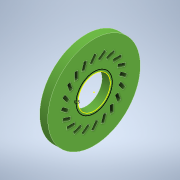
# Autodesk Inventor part: encoder
Saved by Autodesk Inventor 2021 (Build 250183000, 183)
## iProperties
Created: 2021-12-11
Part Number: encoder
Material: Generic
Document SubType Name: Modeling
Designer: Juan M. Casillas
Density: 1 g/cm^3
Appearance: Default
Author: Juan M. Casillas
Autodesk Inventor part; units mm, degrees
ref_plane "YZ Plane" through (0, 0, 0) normal (1, 0, 0) x (0, 1, 0)
ref_plane "XZ Plane" through (0, 0, 0) normal (0, 1, 0) x (-1, 0, 0)
ref_plane "XY Plane" through (0, 0, 0) normal (0, 0, 1) x (1, 0, 0)
sketch "Sketch1" plane through (0, 0, 0) normal (1, 0, 0) x (0, 1, 0)
  circle A0 centre (0, 0) radius 4
  circle A1 centre (0, 0) radius 11.5
  dimension "d0" = 8
  dimension "d1" = 23
  constraints: 2 centre point, 2 coincident
  measures "d0" diameter of A0
  measures "d1" diameter of A1
extrude "Extrusion1" add sketch "Sketch1" along normal mid plane 2
sketch "Sketch2" plane through (1, 0, 0) normal (1, 0, 0) x (0, 0, -1)
  circle A0 centre (0, 0) radius 4 projected
  circle A1 centre (0, 0) radius 4.5
  dimension "d4" = 0.5
  constraints: 1 centre point
  measures "d4" radial gap between concentric circles of A0 A1
sketch "Sketch3" plane through (1, 0, 0) normal (1, 0, 0) x (0, 0, -1)
  circle A0 centre (0, 0) radius 11.5 construction
  circle A1 centre (0, 0) radius 4.5 construction
  line L0 (-4.413, 10.6196) -> (-4.413, 0.8804) construction
  line L1 (-4.813, 6.75) -> (-4.013, 6.75)
  line L2 (-4.013, 6.75) -> (-4.013, 4.75)
  line L3 (-4.013, 4.75) -> (-4.813, 4.75)
  line L4 (-4.813, 4.75) -> (-4.813, 6.75)
  line L5 (-4.813, 6.75) -> (-4.013, 4.75) construction
  line L6 (-4.013, 6.75) -> (-4.813, 4.75) construction
  line L7 (-5.2844, 3.2774) -> (-6.0453, 3.0302)
  line L8 (-6.6633, 4.9323) -> (-5.2844, 3.2774) construction
  line L9 (-5.9025, 5.1795) -> (-6.0453, 3.0302) construction
  line L10 (-6.0453, 3.0302) -> (-6.6633, 4.9323)
  line L11 (-6.6633, 4.9323) -> (-5.9025, 5.1795)
  line L12 (-5.9025, 5.1795) -> (-5.2844, 3.2774)
  line L13 (-6.0386, 1.484) -> (-6.6858, 1.0138)
  line L14 (-7.8614, 2.6318) -> (-6.0386, 1.484) construction
  line L15 (-7.2142, 3.1021) -> (-6.6858, 1.0138) construction
  line L16 (-6.6858, 1.0138) -> (-7.8614, 2.6318)
  line L17 (-7.8614, 2.6318) -> (-7.2142, 3.1021)
  line L18 (-7.2142, 3.1021) -> (-6.0386, 1.484)
  line L19 (-6.2016, -0.4546) -> (-6.6719, -1.1018)
  line L20 (-8.2899, 0.0737) -> (-6.2016, -0.4546) construction
  line L21 (-7.8197, 0.7209) -> (-6.6719, -1.1018) construction
  line L22 (-6.6719, -1.1018) -> (-8.2899, 0.0737)
  line L23 (-8.2899, 0.0737) -> (-7.8197, 0.7209)
  line L24 (-7.8197, 0.7209) -> (-6.2016, -0.4546)
  line L25 (-5.7576, -2.3488) -> (-6.0048, -3.1096)
  line L26 (-7.9069, -2.4916) -> (-5.7576, -2.3488) construction
  line L27 (-7.6597, -1.7308) -> (-6.0048, -3.1096) construction
  line L28 (-6.0048, -3.1096) -> (-7.9069, -2.4916)
  line L29 (-7.9069, -2.4916) -> (-7.6597, -1.7308)
  line L30 (-7.6597, -1.7308) -> (-5.7576, -2.3488)
  line L31 (-4.75, -4.013) -> (-4.75, -4.813)
  line L32 (-6.75, -4.813) -> (-4.75, -4.013) construction
  line L33 (-6.75, -4.013) -> (-4.75, -4.813) construction
  line L34 (-4.75, -4.813) -> (-6.75, -4.813)
  line L35 (-6.75, -4.813) -> (-6.75, -4.013)
  line L36 (-6.75, -4.013) -> (-4.75, -4.013)
  line L37 (-3.2774, -5.2844) -> (-3.0302, -6.0453)
  line L38 (-4.9323, -6.6633) -> (-3.2774, -5.2844) construction
  line L39 (-5.1795, -5.9025) -> (-3.0302, -6.0453) construction
  line L40 (-3.0302, -6.0453) -> (-4.9323, -6.6633)
  line L41 (-4.9323, -6.6633) -> (-5.1795, -5.9025)
  line L42 (-5.1795, -5.9025) -> (-3.2774, -5.2844)
  line L43 (-1.484, -6.0386) -> (-1.0138, -6.6858)
  line L44 (-2.6318, -7.8614) -> (-1.484, -6.0386) construction
  line L45 (-3.1021, -7.2142) -> (-1.0138, -6.6858) construction
  line L46 (-1.0138, -6.6858) -> (-2.6318, -7.8614)
  line L47 (-2.6318, -7.8614) -> (-3.1021, -7.2142)
  line L48 (-3.1021, -7.2142) -> (-1.484, -6.0386)
  line L49 (0.4546, -6.2016) -> (1.1018, -6.6719)
  line L50 (-0.0737, -8.2899) -> (0.4546, -6.2016) construction
  line L51 (-0.7209, -7.8197) -> (1.1018, -6.6719) construction
  line L52 (1.1018, -6.6719) -> (-0.0737, -8.2899)
  line L53 (-0.0737, -8.2899) -> (-0.7209, -7.8197)
  line L54 (-0.7209, -7.8197) -> (0.4546, -6.2016)
  line L55 (2.3488, -5.7576) -> (3.1096, -6.0048)
  line L56 (2.4916, -7.9069) -> (2.3488, -5.7576) construction
  line L57 (1.7308, -7.6597) -> (3.1096, -6.0048) construction
  line L58 (3.1096, -6.0048) -> (2.4916, -7.9069)
  line L59 (2.4916, -7.9069) -> (1.7308, -7.6597)
  line L60 (1.7308, -7.6597) -> (2.3488, -5.7576)
  line L61 (4.013, -4.75) -> (4.813, -4.75)
  line L62 (4.813, -6.75) -> (4.013, -4.75) construction
  line L63 (4.013, -6.75) -> (4.813, -4.75) construction
  line L64 (4.813, -4.75) -> (4.813, -6.75)
  line L65 (4.813, -6.75) -> (4.013, -6.75)
  line L66 (4.013, -6.75) -> (4.013, -4.75)
  line L67 (5.2844, -3.2774) -> (6.0453, -3.0302)
  line L68 (6.6633, -4.9323) -> (5.2844, -3.2774) construction
  line L69 (5.9025, -5.1795) -> (6.0453, -3.0302) construction
  line L70 (6.0453, -3.0302) -> (6.6633, -4.9323)
  line L71 (6.6633, -4.9323) -> (5.9025, -5.1795)
  line L72 (5.9025, -5.1795) -> (5.2844, -3.2774)
  line L73 (6.0386, -1.484) -> (6.6858, -1.0138)
  line L74 (7.8614, -2.6318) -> (6.0386, -1.484) construction
  line L75 (7.2142, -3.1021) -> (6.6858, -1.0138) construction
  line L76 (6.6858, -1.0138) -> (7.8614, -2.6318)
  line L77 (7.8614, -2.6318) -> (7.2142, -3.1021)
  line L78 (7.2142, -3.1021) -> (6.0386, -1.484)
  line L79 (6.2016, 0.4546) -> (6.6719, 1.1018)
  line L80 (8.2899, -0.0737) -> (6.2016, 0.4546) construction
  line L81 (7.8197, -0.7209) -> (6.6719, 1.1018) construction
  line L82 (6.6719, 1.1018) -> (8.2899, -0.0737)
  line L83 (8.2899, -0.0737) -> (7.8197, -0.7209)
  line L84 (7.8197, -0.7209) -> (6.2016, 0.4546)
  line L85 (5.7576, 2.3488) -> (6.0048, 3.1096)
  line L86 (7.9069, 2.4916) -> (5.7576, 2.3488) construction
  line L87 (7.6597, 1.7308) -> (6.0048, 3.1096) construction
  line L88 (6.0048, 3.1096) -> (7.9069, 2.4916)
  line L89 (7.9069, 2.4916) -> (7.6597, 1.7308)
  line L90 (7.6597, 1.7308) -> (5.7576, 2.3488)
  line L91 (4.75, 4.013) -> (4.75, 4.813)
  line L92 (6.75, 4.813) -> (4.75, 4.013) construction
  line L93 (6.75, 4.013) -> (4.75, 4.813) construction
  line L94 (4.75, 4.813) -> (6.75, 4.813)
  line L95 (6.75, 4.813) -> (6.75, 4.013)
  line L96 (6.75, 4.013) -> (4.75, 4.013)
  line L97 (3.2774, 5.2844) -> (3.0302, 6.0453)
  line L98 (4.9323, 6.6633) -> (3.2774, 5.2844) construction
  line L99 (5.1795, 5.9025) -> (3.0302, 6.0453) construction
  line L100 (3.0302, 6.0453) -> (4.9323, 6.6633)
  line L101 (4.9323, 6.6633) -> (5.1795, 5.9025)
  line L102 (5.1795, 5.9025) -> (3.2774, 5.2844)
  line L103 (1.484, 6.0386) -> (1.0138, 6.6858)
  line L104 (2.6318, 7.8614) -> (1.484, 6.0386) construction
  line L105 (3.1021, 7.2142) -> (1.0138, 6.6858) construction
  line L106 (1.0138, 6.6858) -> (2.6318, 7.8614)
  line L107 (2.6318, 7.8614) -> (3.1021, 7.2142)
  line L108 (3.1021, 7.2142) -> (1.484, 6.0386)
  line L109 (-0.4546, 6.2016) -> (-1.1018, 6.6719)
  line L110 (0.0737, 8.2899) -> (-0.4546, 6.2016) construction
  line L111 (0.7209, 7.8197) -> (-1.1018, 6.6719) construction
  line L112 (-1.1018, 6.6719) -> (0.0737, 8.2899)
  line L113 (0.0737, 8.2899) -> (0.7209, 7.8197)
  line L114 (0.7209, 7.8197) -> (-0.4546, 6.2016)
  line L115 (-2.3488, 5.7576) -> (-3.1096, 6.0048)
  line L116 (-2.4916, 7.9069) -> (-2.3488, 5.7576) construction
  line L117 (-1.7308, 7.6597) -> (-3.1096, 6.0048) construction
  line L118 (-3.1096, 6.0048) -> (-2.4916, 7.9069)
  line L119 (-2.4916, 7.9069) -> (-1.7308, 7.6597)
  line L120 (-1.7308, 7.6597) -> (-2.3488, 5.7576)
  point P0 (-4.413, 5.75)
  point P1 (-5.9739, 4.1049)
  point P2 (-6.95, 2.0579)
  point P3 (-7.2458, -0.1905)
  point P4 (-6.8323, -2.4202)
  point P5 (-5.75, -4.413)
  point P6 (-4.1049, -5.9739)
  point P7 (-2.0579, -6.95)
  point P8 (0.1905, -7.2458)
  point P9 (2.4202, -6.8323)
  point P10 (4.413, -5.75)
  point P11 (5.9739, -4.1049)
  point P12 (6.95, -2.0579)
  point P13 (7.2458, 0.1905)
  point P14 (6.8323, 2.4202)
  point P15 (5.75, 4.413)
  point P16 (4.1049, 5.9739)
  point P17 (2.0579, 6.95)
  point P18 (-0.1905, 7.2458)
  point P19 (-2.4202, 6.8323)
  dimension "d7" = 0.8
  dimension "d8" = 2
  dimension "d11" = 360
  constraints: 242 end point, 41 midpoint, 2 parallel, 1 coincident, 1 horizontal, 1 perpendicular, 1 vertical, 225 other
  measures "d7" distance of L2.end L3.end
  measures "d8" distance of L1.end L2.end
extrude "Extrusion3" cut sketch "Sketch3" against normal blind 5
body "Solid1"
